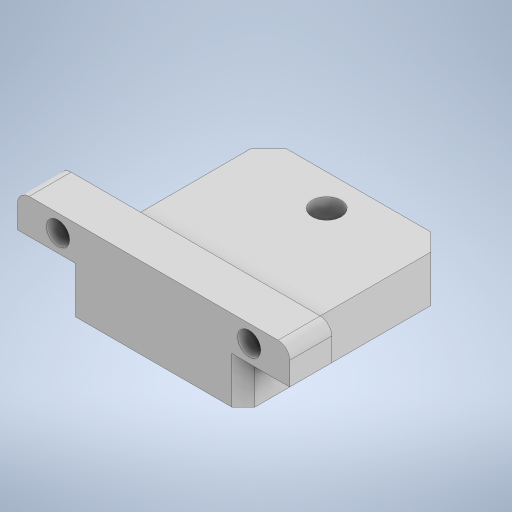
# Autodesk Inventor part: camera_holder
Saved by Autodesk Inventor 2024 (Build 280153000, 153)
## iProperties
Created: 2024-07-17
Part Number: camera_holder
Material: Generic
Document SubType Name: Modeling
Designer: mamof
Density: 1 g/cm^3
Appearance: Default
Author: mamof
Autodesk Inventor part; units mm, degrees
ref_plane "YZ Plane" through (0, 0, 0) normal (1, 0, 0) x (0, 1, 0)
ref_plane "XZ Plane" through (0, 0, 0) normal (0, 1, 0) x (-1, 0, 0)
ref_plane "XY Plane" through (0, 0, 0) normal (0, 0, 1) x (1, 0, 0)
sketch "Sketch1" plane through (0, 0, 0) normal (0, 1, 0) x (-1, 0, 0)
  line L0 (29, 0) -> (31, -2)
  line L1 (28, -35.353) -> (31, -32.353)
  line L2 (0, -32.353) -> (3, -35.353)
  line L3 (0, -2) -> (2, 0)
  line L4 (31, -2) -> (31, -32.353)
  line L5 (28, -35.353) -> (3, -35.353)
  line L6 (0, -32.353) -> (0, -2)
  line L7 (2, 0) -> (29, 0)
  point P0 (0, 0)
  dimension "d5" = 2
  dimension "d6" = 2
  constraints: 16 end point, 3 perpendicular, 1 vertical
  measures "d5" distance of point (0, 0) L3.end
  measures "d6" distance of point (0, 0) L3.start
extrude "Extrusion1" add sketch "Sketch1" along normal blind 8
sketch "Sketch2" plane through (0, 0, -2) normal (1, 0, 0) x (0, 0, -1)
  line L0 (0, 0) -> (0, 8) projected
  line L1 (0, 8) -> (8.207, 8)
  line L2 (30.353, 8) -> (0, 8) projected
  line L3 (8.207, 8) -> (8.207, 5)
  circle A0 centre (8.207, 5) radius 1.6
  point P0 (-2, 0)
  dimension "d13" = 8.207
  dimension "d14" = 3
  dimension "d15" = 3.2
  constraints: 4 end point, 1 centre point, 1 coincident, 1 point on line, 1 vertical
  measures "d13" distance of L0.end L1.end
  measures "d14" distance of L1.end L3.end
  measures "d15" diameter of A0
extrude "Extrusion2" cut sketch "Sketch2" against normal blind 31
sketch "Sketch3" plane through (0, 8, 0) normal (0, 1, 0) x (1, 0, 0)
  line L0 (-31, 2) -> (-29, 0) projected
  line L1 (-29, 0) -> (-39, 0)
  line L2 (-2, 0) -> (0, 2) projected
  line L3 (-2, 0) -> (8, 0)
  line L4 (-39, 0) -> (-39, 14.511)
  line L5 (8, 0) -> (8, 14.511)
  line L6 (8, 14.511) -> (-39, 14.511)
  line L7 (-29, 0) -> (-2, 0)
  point P0 (0, 0)
  dimension "d18" = 10
  dimension "d19" = 10
  dimension "d20" = 14.511
  dimension "d21" = 14.511
  constraints: 12 end point, 3 horizontal, 2 vertical
  measures "d18" distance of L0.end L1.end
  measures "d19" distance of L2.start L3.end
  measures "d20" distance of L1.end L4.end
  measures "d21" distance of L3.end L5.end
extrude "Extrusion3" add sketch "Sketch3" along normal blind 6
sketch "Sketch4" plane through (-29, 0, 0) normal (0, 0, 1) x (1, 0, 0)
  line L0 (-10, 14) -> (37, 14) projected
  line L1 (37, 14) -> (35, 14)
  line L2 (35, 14) -> (35, 12)
  circle A0 centre (35, 12) radius 2
  line L3 (-10, 8) -> (-10, 14) projected
  line L4 (-10, 14) -> (-8, 14)
  line L5 (-8, 14) -> (-8, 12)
  circle A1 centre (-8, 12) radius 2
  line L6 (-10, 14) -> (-10, 12)
  line L7 (37, 14) -> (37, 12)
  line L8 (37, 8) -> (37, 14) projected
  point P0 (29, 0)
  point P1 (-8, 14)
  dimension "d26" = 4
  dimension "d29" = 4
  dimension "d24" = 2
  dimension "d25" = 2
  dimension "d27" = 2
  dimension "d28" = 2
  constraints: 12 end point, 4 point on line, 2 coincident, 2 perpendicular, 6 other
  measures "d24" distance of L0.end L1.end
  measures "d25" distance of L1.end L2.end
  measures "d27" distance of L0.start L4.end
  measures "d28" distance of L4.end L5.end
extrude "Extrusion4" cut sketch "Sketch4" against normal blind 14.511 contours L0 L7 A0 | L0 A1 L3
sketch "Sketch5" plane through (-29, 0, 0) normal (0, 0, 1) x (1, 0, 0)
  arc A0 (37, 12) -> (35, 14) centre (35, 12) ccw projected
  line L0 (35, 14) -> (30, 14)
  line L1 (35, 14) -> (-8, 14) projected
  line L2 (30, 14) -> (30, 11)
  line L3 (-8, 14) -> (-3, 14)
  line L4 (-3, 14) -> (-3, 11)
  circle A1 centre (-3, 11) radius 2
  circle A2 centre (30, 11) radius 2
  point P0 (29, 0)
  dimension "d32" = 5
  dimension "d33" = 3
  dimension "d34" = 5
  dimension "d35" = 3
  dimension "d36" = 4
  dimension "d37" = 4
  constraints: 8 end point, 2 centre point, 2 coincident, 2 perpendicular, 2 point on line
  measures "d32" distance of L0.start L0.end
  measures "d33" distance of L0.end L2.end
  measures "d34" distance of L1.end L3.end
  measures "d35" distance of L3.end L4.end
  measures "d36" diameter of A1
  measures "d37" diameter of A2
extrude "Extrusion5" cut sketch "Sketch5" against normal blind 14.511
sketch "Sketch6" plane through (0, 8, 0) normal (0, 1, 0) x (1, 0, 0)
  line L0 (-28, 35.353) -> (-31, 32.353) projected
  line L1 (-28, 35.353) -> (-28, 24.409)
  line L2 (0, 32.353) -> (-3, 35.353) projected
  line L3 (-3, 35.353) -> (-3, 24.409)
  line L4 (-3, 24.409) -> (-28, 24.409)
  line L5 (-28, 35.353) -> (-3, 35.353)
  line L6 (-3, 35.353) -> (-28, 35.353) projected
  line L7 (-28, 35.353) -> (-15.5, 35.353)
  line L8 (-15.5, 35.353) -> (-15.5, 29.881)
  circle A0 centre (-15.5, 29.881) radius 2.5
  point P0 (0, 0)
  dimension "d40" = 10.944
  dimension "d41" = 10.944
  dimension "d42" = 12.5
  dimension "d43" = 5.472
  dimension "d44" = 5
  constraints: 12 end point, 3 vertical, 1 centre point, 1 coincident, 1 midpoint
  measures "d40" distance of L0.start L1.end
  measures "d41" distance of L2.end L3.end
  measures "d42" distance of L0.start L7.end
  measures "d43" distance of L7.end L8.end
  measures "d44" diameter of A0
extrude "Extrusion6" cut sketch "Sketch6" against normal blind 8 contours A0
sketch "Sketch7" plane through (8, 8, -14.511) normal (0, 0, -1) x (-1, 0, 0)
  line L0 (0, 0) -> (8, 0) projected
  line L1 (47, 0) -> (47, 4) projected
  line L2 (0, 0) -> (47, 0)
  line L3 (47, 0) -> (47, 6)
  line L4 (47, 6) -> (0, 6)
  line L5 (0, 6) -> (0, 0)
  point P0 (8, -8)
  dimension "d47" = 6
  dimension "d48" = 47
  constraints: 8 end point, 2 perpendicular, 1 horizontal
  measures "d47" distance of L1.start L3.end
  measures "d48" distance of L3.end L4.end
extrude "Extrusion7" cut sketch "Sketch7" against normal blind 7.2555
body "Solid1"
